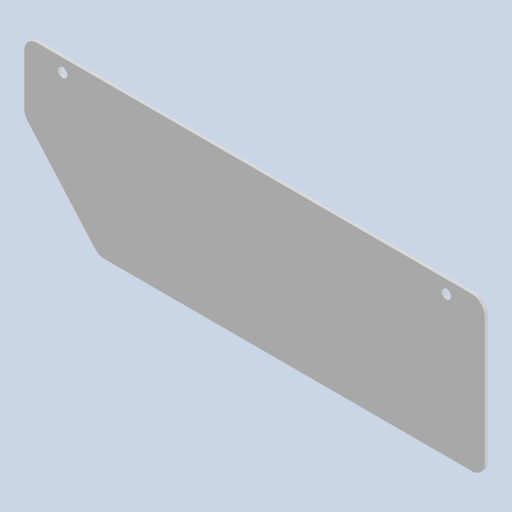
# Autodesk Inventor part: wingpoly
Saved by Autodesk Inventor 2024.2 (Build 282272000, 272)
## iProperties
Created: 2023-12-27
Part Number: wingpoly
Material: Generic
Document SubType Name: Sheet Metal
Designer: reima
Density: 1 g/cm^3
Sheet Metal Rule: Default
Appearance: Default
Flat Pattern Width: 7.62 cm
Flat Pattern Length: 22.86 cm
Flat Pattern Area: 174.193 cm^2
Sheet Metal Width: 3.000 in
Sheet Metal Length: 9.000 in
Sheet Metal Area: 27.000 in^2
Author: reima
Autodesk Inventor part; units mm, degrees
ref_plane "YZ Plane" through (0, 0, 0) normal (1, 0, 0) x (0, 1, 0)
ref_plane "XZ Plane" through (0, 0, 0) normal (0, 1, 0) x (-1, 0, 0)
ref_plane "Work Plane1" through (0, 0, 0) normal (0, 0, 1) x (1, 0, 0)
sketch "Sketch1" plane through (0, 0, 0) normal (0, 0, 1) x (1, 0, 0)
  circle A0 centre (228.1, 21.9203) radius 2.3114
  circle A1 centre (431.3, 21.9203) radius 2.3114
  line L0 (318.0242, 34.6203) -> (379.4758, 34.6203)
  line L1 (215.4, 19.6089) -> (215.4, 11.6079)
  line L2 (444, 9.2203) -> (444, 11.6079)
  line L3 (221.75, 34.6203) -> (437.65, 34.6203)
  line L4 (444, 28.2703) -> (444, -35.2297)
  line L5 (437.65, -41.5797) -> (255.2197, -41.5797)
  line L6 (215.4, 3.0597) -> (215.4, 28.2703)
  line L7 (190.0994, 1.6338) -> (231.0454, -48.1215) construction
  arc A2 (437.65, -41.5797) -> (444, -35.2297) centre (437.65, -35.2297) ccw
  arc A3 (221.75, 34.6203) -> (215.4, 28.2703) centre (221.75, 28.2703) ccw
  arc A4 (444, 28.2703) -> (437.65, 34.6203) centre (437.65, 28.2703) ccw
  line L8 (218.8779, -3.3569) -> (250.4419, -39.4124)
  line L9 (218.8779, -3.3569) -> (216.9197, -1.0623)
  arc A5 (250.4419, -39.4124) -> (255.2197, -41.5797) centre (255.2197, -35.2297) ccw
  arc A6 (215.4, 3.0597) -> (216.9197, -1.0623) centre (221.75, 3.0597) ccw
  point P0 (0, 0)
  point P1 (444, -41.5797)
  point P2 (444, 34.6203)
  point P3 (444, 10.4141)
  point P4 (215.4, 15.6084)
  point P5 (379.4758, 34.6203)
  point P6 (252.3392, -41.5797)
  dimension "d0" = 76.2
  dimension "d1" = 0
  dimension "d3" = 0
  dimension "d5" = 6.35
  dimension "d6" = 6.35
  dimension "d19" = 50.8
  dimension "d21" = 6.35
  measures "d0" distance of point (444, 34.62) point (444, -41.58)
  measures "d1" distance from line of point (444, 10.414) L4
  measures "d3" distance between parallel lines of L0 L3
  measures "d5" radius of A2
  measures "d6" radius of A3
  measures "d19" distance of L8.start point (252.339, -41.58)
  measures "d21" radius of A5
extrude "Plate1" add sketch "Sketch1" along normal blind 1.5875
sketch "Sketch5" plane through (221.75, 34.6203, 1.5875) normal (0, 0, 1) x (1, 0, 0)
  circle A0 centre (6.35, -12.7) radius 2.3114 projected
  circle A1 centre (12.7, -6.35) radius 2.3368
  circle A2 centre (19.05, -12.7) radius 1.5652 construction
  point P0 (-221.75, -34.6203)
  dimension "d22" = 4.6736
  dimension "d31" = 12.7
  dimension "d32" = 6.35
  dimension "d33" = -6.35
  constraints: 2 centre point
  measures "d22" diameter of A1
  measures "d31" distance of A2.centre A0.centre
  measures "d32" horizontal distance of A2.centre A1.centre
  measures "d33" horizontal distance of A2.centre A1.centre
sheet face with bend "Face2" sketch "Sketch5" thickness 1.5875 toward (0, 0, -1) bend radius 1.5875 contours A0
bend "Bend1"
extrude "Cut1" cut sketch "Sketch5" against normal blind 1.5875 contours A1
sketch "Sketch6" plane through (0, 0, 1.5875) normal (0, 0, 1) x (1, 0, 0)
  circle A0 centre (424.95, 28.2703) radius 2.3368
  circle A1 centre (418.6, 21.9203) radius 1.1969 construction
  circle A2 centre (431.3, 21.9203) radius 2.3114 projected
  point P0 (0, 0)
  dimension "d34" = 4.6736
  dimension "d35" = 6.35
  dimension "d36" = 0
  dimension "d37" = 12.7
  dimension "d38" = 6.35
  constraints: 2 centre point
  measures "d34" diameter of A0
  measures "d35" horizontal distance of A1.centre A0.centre
  measures "d36" vertical distance of A2.centre A1.centre
  measures "d37" distance of A2.centre A1.centre
  measures "d38" horizontal distance of A1.centre A0.centre
sheet face with bend "Face3" sketch "Sketch6" thickness 1.5875 toward (0, 0, -1) bend radius 1.5875 contours A2
bend "Bend2"
extrude "Cut2" cut sketch "Sketch6" against normal blind 1.5875 contours A0
equation "\"d29\" = Thickness"
equation "\"d44\" = Thickness"
equation "\"d7\" = Thickness"
equation "\"d24\" = BendRadius"
equation "\"d25\" = BendReliefWidth"
equation "\"d27\" = MinimumRemnant"
equation "\"d26\" = BendReliefDepth"
equation "\"d28\" = TransitionRadius"
equation "\"d39\" = BendRadius"
equation "\"d40\" = BendReliefWidth"
equation "\"d42\" = MinimumRemnant"
equation "\"d41\" = BendReliefDepth"
equation "\"d43\" = TransitionRadius"
equation "\"BendRadius\" = Thickness"
equation "\"BendReliefWidth\" = Thickness"
equation "\"BendReliefDepth\" = 0.5 * Thickness"
equation "\"CornerReliefSize\" = 4 * Thickness"
equation "\"MinimumRemnant\" = 2 * Thickness"
equation "\"TransitionRadius\" = BendRadius"
equation "\"JacobiRadiusSize\" = BendRadius"
equation "\"GapSize\" = Thickness"
equation "\"Thickness\" = 1.5875"
body "Solid1"
